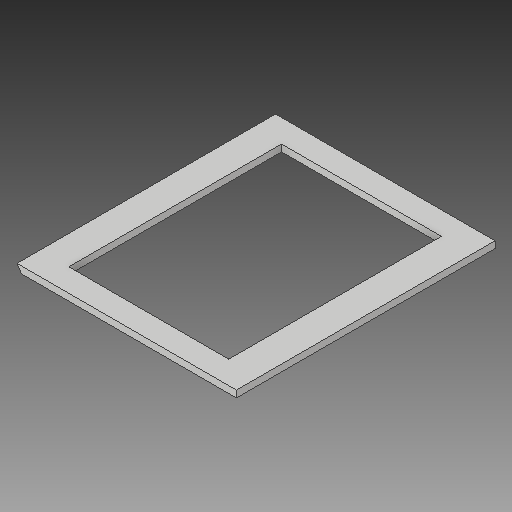
# Autodesk Inventor part: screen_holder
Saved by Autodesk Inventor 2017 (Build 210142000, 142)
## iProperties
Created: 2019-03-22
Part Number: screen_holder
Material: Generic
Document SubType Name: Modeling
Designer: Mitch
Density: 1 g/cm^3
Appearance: Default
Author: Mitch
Autodesk Inventor part; units mm, degrees
ref_plane "YZ Plane" through (0, 0, 0) normal (1, 0, 0) x (0, 1, 0)
ref_plane "XZ Plane" through (0, 0, 0) normal (0, 1, 0) x (-1, 0, 0)
ref_plane "XY Plane" through (0, 0, 0) normal (0, 0, 1) x (1, 0, 0)
sketch "Sketch1" plane through (0, 0, 0) normal (0, 1, 0) x (-1, 0, 0)
  line L0 (0, 0) -> (204.7875, 0)
  line L1 (204.7875, 0) -> (204.7875, -241.3)
  line L2 (204.7875, -241.3) -> (0, -241.3)
  line L3 (0, -241.3) -> (0, 0)
  dimension "d0" = 204.7875
  dimension "d1" = 241.3
  constraints: 8 end point, 2 parallel, 1 horizontal, 1 perpendicular
  measures "d0" distance of L1.end L2.end
  measures "d1" distance of L0.end L1.end
extrude "Extrusion1" add sketch "Sketch1" along normal blind 6.35
sketch "Sketch2" plane through (0, 6.35, 0) normal (0, 1, 0) x (1, 0, 0)
  line L0 (-28.575, 219.8688) -> (-177.8, 219.8688)
  line L1 (-177.8, 219.8688) -> (-177.8, 21.4312)
  line L2 (-177.8, 21.4312) -> (-28.575, 21.4313)
  line L3 (-28.575, 21.4313) -> (-28.575, 219.8688)
  line L4 (0, 0) -> (-204.7875, 0) projected
  line L5 (-204.7875, 241.3) -> (-204.7875, 0) projected
  dimension "d4" = 149.225
  dimension "d5" = 198.4375
  dimension "d6" = 21.4312
  dimension "d7" = 26.9875
  constraints: 8 end point, 2 parallel, 1 horizontal, 1 perpendicular
  measures "d4" distance of L2.end L1.end
  measures "d5" distance of L2.end L0.start
  measures "d6" distance between parallel lines of L4 L2
  measures "d7" distance between parallel lines of L5 L1
extrude "Extrusion2" cut sketch "Sketch2" against normal blind 25.4
sketch "Sketch4" plane through (-204.7875, 0, 0) normal (0, 0, 1) x (1, 0, 0)
  line L0 (4.2831, 0) -> (-0.0504, 6.4246) projected
  line L1 (0, 0) -> (0, 6.35) projected
  line L2 (204.7875, 0) -> (0, 0) projected
  line L3 (0, 6.35) -> (0, 0)
  line L4 (0, 0) -> (4.2831, 0)
  constraints: 4 end point, 2 point on line, 1 vertical
extrude "Extrusion4" cut sketch "Sketch4" against normal blind 241.3
body "Solid1"
